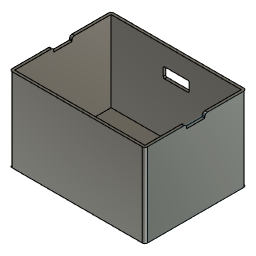
Button Case (Autodesk Fusion 360 design; units mm, degrees)
Autodesk Fusion 360 part; units mm, degrees
note: some values were not read from the file. Chosen so that the rebuilt part matches the saved one: which face or edge a step refers to.
sketch "Sketch1" plane through (0, 0, 0) normal (0, 0, 1) x (1, 0, 0)
  line L0 (1, 0) -> (51, 0)
  line L1 (52, 1) -> (52, 38)
  line L2 (51, 39) -> (1, 39)
  line L3 (0, 38) -> (0, 1)
  arc A0 (1, 39) -> (0, 38) centre (1, 38) ccw
  arc A1 (52, 38) -> (51, 39) centre (51, 38) ccw
  arc A2 (51, 0) -> (52, 1) centre (51, 1) ccw
  arc A3 (0, 1) -> (1, 0) centre (1, 1) ccw
  point P0 (52, 0)
  point P1 (0, 39)
  dimension "d1" = 52
  dimension "d2" = 39
  dimension "d3" = 1
  constraint horizontal L0
  constraint vertical L1
  constraint horizontal L2
  constraint vertical L3
  constraint coincident P1 L2
  constraint coincident P1 L3
  constraint tangent L2 A0
  constraint tangent L3 A0
  constraint tangent L1 A1
  constraint tangent L2 A1
  constraint equal A0 A1
  constraint coincident P0 L0
  constraint coincident P0 L1
  constraint tangent L0 A2
  constraint tangent L1 A2
  constraint equal A0 A2
  constraint coincident origin L0
  constraint coincident origin L3
  constraint tangent L0 A3
  constraint tangent L3 A3
  constraint equal A0 A3
  measures "d1" distance of origin P0
  measures "d2" distance of origin P1
  measures "d3" radius of A0
extrude "Extrude1" add sketch "Sketch1" along normal blind 30
sketch "Sketch2" plane through (0, 0, 30) normal (0, 0, 1) x (-1, 0, 0)
  arc A0 (0, -1) -> (-1, 0) centre (-1, -1) ccw
  line L0 (-1, 0) -> (-51, 0)
  arc A1 (-51, 0) -> (-52, -1) centre (-51, -1) ccw
  line L1 (-52, -1) -> (-52, -38)
  arc A2 (-52, -38) -> (-51, -39) centre (-51, -38) ccw
  line L2 (-51, -39) -> (-1, -39)
  arc A3 (-1, -39) -> (0, -38) centre (-1, -38) ccw
  line L3 (0, -38) -> (0, -1)
  line L4 (-1, -38) -> (-1, -1)
  line L5 (-1, -1) -> (-51, -1)
  line L6 (-51, -1) -> (-51, -38)
  line L7 (-51, -38) -> (-1, -38)
  dimension "d6" = -1
extrude "Extrude2" cut sketch "Sketch2" against normal blind 29 contours L4 L5 L6 L7
sketch "Sketch3" plane through (52, 0, 0) normal (1, 0, 0) x (0, 1, 0)
  line L0 (1, 0) -> (38, 0)
  line L1 (38, 0) -> (38, 30)
  line L2 (38, 30) -> (1, 30)
  line L3 (1, 30) -> (1, 0)
  line L4 (16, 30) -> (23, 30)
  line L5 (23, 30) -> (23, 28.5)
  line L6 (23, 28.5) -> (16, 28.5)
  line L7 (16, 28.5) -> (16, 30)
  dimension "d9" = 7
  dimension "d10" = 1.5
  dimension "d11" = 15
  constraint horizontal L4
  constraint vertical L5
  constraint horizontal L6
  constraint vertical L7
  constraint coincident L2 L4.start
  measures "d9" distance of L4.start L4.end
  measures "d10" distance of L4.start L6.end
  measures "d11" distance of L3 L7
extrude "Extrude3" cut sketch "Sketch3" against normal blind 50 contours L2 L4 L5 L6 L7
fillet "Fillet1" radius 1 4 edges at (51.5, 16, 30) (51.5, 23, 30) (51.5, 16, 30) (51.5, 23, 30)
sketch "Sketch4" plane through (0, 39, 0) normal (0, 1, 0) x (-1, 0, 0)
  line L0 (-51, 0) -> (-1, 0)
  line L1 (-1, 0) -> (-1, 30)
  line L2 (-1, 30) -> (-51, 30)
  line L3 (-51, 30) -> (-51, 0)
  line L4 (-30.5, 24.8677) -> (-21.5, 24.8677)
  line L5 (-21, 24.3677) -> (-21, 21.3677)
  line L6 (-21.5, 20.8677) -> (-30.5, 20.8677)
  line L7 (-31, 21.3677) -> (-31, 24.3677)
  arc A0 (-30.5, 24.8677) -> (-31, 24.3677) centre (-30.5, 24.3677) ccw
  arc A1 (-31, 21.3677) -> (-30.5, 20.8677) centre (-30.5, 21.3677) ccw
  arc A2 (-21.5, 20.8677) -> (-21, 21.3677) centre (-21.5, 21.3677) ccw
  arc A3 (-21, 24.3677) -> (-21.5, 24.8677) centre (-21.5, 24.3677) ccw
  point P0 (-31, 24.8677)
  point P1 (-21, 24.8677)
  point P2 (-31, 20.8677)
  dimension "d16" = 10
  dimension "d17" = 4
  dimension "d18" = 20
  dimension "d19" = 0.5
  constraint horizontal L4
  constraint vertical L5
  constraint horizontal L6
  constraint vertical L7
  constraint coincident P0 L4
  constraint coincident P0 L7
  constraint tangent L4 A0
  constraint tangent L7 A0
  constraint coincident P2 L6
  constraint coincident P2 L7
  constraint tangent L6 A1
  constraint tangent L7 A1
  constraint equal A0 A1
  constraint tangent L5 A2
  constraint tangent L6 A2
  constraint equal A0 A2
  constraint coincident P1 L4
  constraint coincident P1 L5
  constraint tangent L4 A3
  constraint tangent L5 A3
  constraint equal A0 A3
  measures "d16" distance of P0 P1
  measures "d17" distance of P0 P2
  measures "d18" distance of L3 L7
  measures "d19" radius of A0
extrude "Extrude4" cut sketch "Sketch4" against normal blind 1 contours L4 L5 L6 L7 A0 A1 A2 A3
extrude "Extrude5" cut sketch "Sketch3" against normal blind 55 contours L2 L4 L5 L6 L7
fillet "Fillet2" radius 1 2 edges at (0.5, 23, 30) (0.5, 16, 30)
delete_face "DeleteFace1" 1 faces at (51.6667, 23.0181, 29.1893)
delete_face "DeleteFace2" 1 faces at (0.6667, 23.0181, 29.1893)
delete_face "DeleteFace3" 1 faces at (51.6667, 15.8888, 29.4582)
delete_face "DeleteFace4" 1 faces at (0.6667, 15.8888, 29.4582)
delete_face "DeleteFace5" 3 faces at (0.3333, 23, 29) (0.6667, 20.6667, 28.5) (0.6667, 16, 29)
delete_face "DeleteFace6" 3 faces at (51.6667, 23, 29.5) (51.6667, 20.6667, 28.5) (51.6667, 16, 29)
move_face "OffsetFaces1" offset 1 1 faces at (34.3333, 0.3333, 30)
move_face "OffsetFaces2" offset 1 1 faces at (34.3333, 0.3333, 31)
sketch "Sketch5" plane through (52, 0, 0) normal (1, 0, 0) x (0, 1, 0)
  line L0 (38, 32) -> (1, 32)
  line L1 (1, 32) -> (1, 0)
  line L2 (1, 0) -> (38, 0)
  line L3 (38, 0) -> (38, 32)
sketch "Sketch6" plane through (52, 0, 0) normal (1, 0, 0) x (0, 1, 0)
  line L0 (16, 32) -> (23, 32)
  line L1 (23, 32) -> (23, 30.5)
  line L2 (23, 30.5) -> (16, 30.5)
  line L3 (16, 30.5) -> (16, 32)
  line L4 (1, 32) -> (1, 0)
  line L5 (38, 32) -> (1, 32)
  dimension "d28" = 7
  dimension "d29" = 1.5
  dimension "d30" = 15
  constraint horizontal L0
  constraint vertical L1
  constraint horizontal L2
  constraint vertical L3
  constraint collinear L0 L5
  measures "d28" distance of L0.start L0.end
  measures "d29" distance of L0.start L2.end
  measures "d30" distance of L3 L4
extrude "Extrude6" cut sketch "Sketch6" against normal blind 54
fillet "Fillet3" radius 1 4 edges at (51.5, 23, 32) (51.5, 16, 32) (0.5, 16, 32) (0.5, 23, 32)
